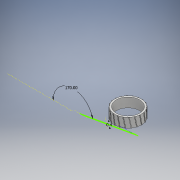
# Autodesk Inventor part: net2
Saved by Autodesk Inventor 2018 (Build 220112000, 112)
## iProperties
Created: 2019-09-09
Part Number: net2
Material: Generic
Document SubType Name: Modeling
Designer: dsikar
Density: 1 g/cm^3
Appearance: Default
Author: dsikar
Autodesk Inventor part; units mm, degrees
ref_plane "YZ Plane" through (0, 0, 0) normal (1, 0, 0) x (0, 1, 0)
ref_plane "XY Plane" through (0, 0, 0) normal (0, 0, 1) x (1, 0, 0)
sketch "Sketch1" plane through (0, 0, 0) normal (0, 1, 0) x (-1, 0, 0)
  line L0 (8.7, 0) -> (9.9, 0)
  line L1 (9.9, 0) -> (9.9, 7)
  line L2 (9.9, 7) -> (8.7, 7)
  line L3 (8.7, 7) -> (8.7, 0)
  line L4 (0, -1.4) -> (0, 8.4) projected
  point P0 (0, 0)
  dimension "d0" = 1.2
  dimension "d1" = 7
  dimension "d2" = 8.7
  constraints: 8 end point, 2 parallel, 1 horizontal, 1 perpendicular
  measures "d0" distance of L2.end L1.end
  measures "d1" distance of L1.end L0.end
  measures "d2" distance from line of L3 point (0, 0)
revolve "Revolution1" add sketch "Sketch1" angle 360 about axis through (0, 0, -10) along (0, 0, 1)
ref_plane "Work Plane1" through (0, -15.5, 0) normal (0, 1, 0) x (-1, 0, 0)
sketch "Sketch8" plane through (0, -15.5, 0) normal (0, 1, 0) x (-1, 0, 0)
  line L0 (0, 0) -> (1.2343, 7)
  line L1 (0, 0) -> (7.8694, 0) construction
  line L2 (0.8281, 7) -> (-0.4062, 0)
  line L3 (1.2316, 6.985) -> (0.8281, 7)
  line L4 (-9.9, 7) -> (9.9, 7) projected
  line L5 (0, 0) -> (-0.4062, 0)
  line L6 (-9.9, 0) -> (9.9, 0) projected
  dimension "d19" = 80
  dimension "d20" = 0.4
  constraints: 10 end point, 4 point on line, 1 horizontal
  measures "d19" angle of L1 L0
  measures "d20" distance between parallel lines of L0 L2
emboss "Emboss3" sketch "Sketch8" operation add depth 0.3 direction (0, -1, 0) wrap yes faces at (-9.7718, 1.5881, 2.3333) contours L5 L2 L3 L0
pattern_circular "Circular Pattern2" count 20 over 360 about axis through (0, 0, 3.5) along (0, 0, -1) of "Emboss3"
sketch "Sketch9" plane through (0, -15.5, 0) normal (0, 1, 0) x (-1, 0, 0)
  line L0 (18.3768, 0) -> (-21.3222, 7)
  line L1 (25.6566, -1.2836) -> (75.1217, -1.2836) construction
  line L2 (-19.0187, 7) -> (20.6803, 0)
  line L3 (-9.1269, 7) -> (-7.4951, 7) construction
  line L4 (8.0093, 0) -> (9.2821, 0) construction
  line L5 (18.3768, 0) -> (20.6803, 0)
  line L6 (-8.4715, 7) -> (-23.5513, 7) construction
  line L7 (-16.7152, 7) -> (-21.3222, 7) construction
  line L8 (24.9077, 0) -> (14.8317, 0) construction
  line L9 (20.6803, 0) -> (18.3471, 0) construction
  line L10 (-18.9778, 7) -> (-19.0187, 7)
  line L11 (-21.2863, 7) -> (-21.3222, 7)
  line L12 (-17.5714, 6.7448) -> (-20.6595, 7.3051)
  line L13 (-20.0494, 6.7756) -> (-22.8834, 7.2898)
  line L14 (-20.575, 7.2898) -> (-22.8834, 7.2898)
  line L15 (-18.9778, 7) -> (-19.0187, 7)
  line L16 (-21.2863, 7) -> (-21.3222, 7)
  line L17 (-18.9778, 7) -> (-19.0187, 7)
  line L18 (-21.2863, 7) -> (-21.3222, 7)
  dimension "d26" = 170
  dimension "d27" = 0.4
  constraints: 34 end point, 15 point on line, 5 horizontal, 3 collinear, 1 midpoint, 1 parallel, 1 other
  measures "d26" angle of L1 L0
  measures "d27" distance between parallel lines of L0 L2
body "Solid1"
